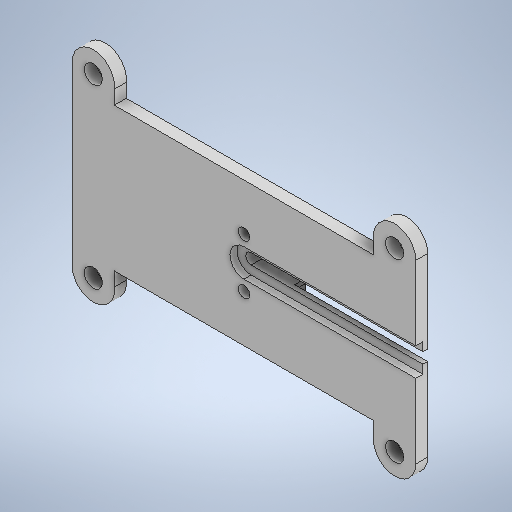
# Autodesk Inventor part: Gripper_BackPlate
Saved by Autodesk Inventor 2025.1 (Build 291241000, 241)
## iProperties
Created: 2024-08-02
Part Number: Gripper_BackPlate
Material: Generic
Document SubType Name: Modeling
Designer: leonh
Density: 1 g/cm^3
Appearance: Default
Author: leonh
Autodesk Inventor part; units mm, degrees
ref_plane "YZ Plane" through (0, 0, 0) normal (1, 0, 0) x (0, 1, 0)
ref_plane "XZ Plane" through (0, 0, 0) normal (0, 1, 0) x (-1, 0, 0)
ref_plane "XY Plane" through (0, 0, 0) normal (0, 0, 1) x (1, 0, 0)
sketch "Sketch1" plane through (0, 0, 0) normal (0, 0, 1) x (1, 0, 0)
  line L0 (-8.76, 11.0126) -> (-8.76, 0.5126)
  line L1 (-8.76, 0.5126) -> (-11.24, -14.9874)
  line L2 (-11.24, -14.9874) -> (8.76, -14.9874)
  line L3 (8.76, -14.9874) -> (8.76, -4.4874)
  line L4 (11.24, 11.0126) -> (-8.76, 11.0126)
  line L5 (0, 12.916) -> (0, -18.5653)
  line L6 (-8.76, 0.5126) -> (13.6474, 0.5126) construction
  line L7 (8.76, -4.4874) -> (-2.6872, -4.4874) construction
  line L8 (-5.8361, -1.9874) -> (18.6079, -1.9874) construction
  circle A0 centre (0, -7.7374) radius 1.325
  circle A1 centre (0, 3.7626) radius 1.325
  line L9 (22.7948, -1.9874) -> (0, -1.9874) construction
  line L10 (9.36, -0.7374) -> (0, -0.7374)
  line L11 (0, -3.2374) -> (8.96, -3.2374)
  arc A2 (0, -0.7374) -> (0, -3.2374) centre (0, -1.9874) ccw
  line L12 (8.76, -4.4874) -> (8.96, -3.2374)
  line L13 (9.36, -0.7374) -> (11.24, 11.0126)
  point P0 (0, 0)
  point P1 (-8.76, -4.4874)
  point P2 (11.3974, -1.9874)
  dimension "d0" = 2.48
  dimension "d1" = 15.5
  dimension "d2" = 15.5
  dimension "d3" = 2.48
  dimension "d4" = 10.5
  dimension "d5" = 10.5
  dimension "d6" = 20
  dimension "d7" = 20
  dimension "d8" = 2.65
  dimension "d9" = 7.25
  dimension "d12" = 2.5
  dimension "d26" = 11.75
  dimension "d27" = 14.25
  constraints: 30 end point, 4 point on line, 3 centre point, 2 horizontal, 2 perpendicular, 2 point on circle, 2 symmetric about line, 2 tangent, 2 vertical, 2 vertical alignment, 1 collinear, 1 midpoint, 1 parallel, 2 other
  measures "d0" horizontal distance of L1.end L0.end
  measures "d1" vertical distance of L1.end L0.end
  measures "d2" vertical distance of L4.start L3.end
  measures "d3" horizontal distance of L4.start L3.end
  measures "d4" distance of L0.start L0.end
  measures "d5" distance of L2.end L3.end
  measures "d6" distance of L4.start L0.start
  measures "d7" distance of L2.end L1.end
  measures "d8" diameter of A0
  measures "d9" distance from line of A0.centre L2
  measures "d12" diameter of A2
  measures "d26" vertical distance of L2.end L11.end
  measures "d27" vertical distance of L2.end L10.start
extrude "Extrusion1" add sketch "Sketch1" against normal blind 2.8 contours L4 L5 A1 A2 A0 L2 L1 L0 | L4 L13 L10 L5 A1 | L5 A0 L11 L12 L3 L2
sketch "Sketch2" plane through (0, 0, 0) normal (0, 0, 1) x (1, 0, 0)
  line L0 (-39.75, -18.5874) -> (-39.75, 14.6126)
  line L1 (0, 12.916) -> (0, -18.5653) construction
  line L2 (-5.8361, -1.9874) -> (18.6079, -1.9874) construction
  line L3 (-39.75, 14.6126) -> (-39.75, 18.4126)
  line L4 (-29.9847, 14.6126) -> (-29.9847, 17.8301)
  arc A0 (-29.9847, 17.8301) -> (-39.75, 18.4126) centre (-34.85, 18.4126) ccw
  line L5 (0, 12.916) -> (0, -18.5653)
  circle A1 centre (-34.85, 18.4126) radius 2.1
  arc A2 (0, -0.7374) -> (0, -3.2374) centre (0, -1.9874) ccw projected
  line L6 (-1.25, -1.9874) -> (17.7749, -1.9874) construction
  line L7 (0, -3.2374) -> (39.75, -3.2374)
  line L8 (39.75, -0.7374) -> (0, -0.7374)
  arc A3 (0, -0.7374) -> (0, -3.2374) centre (0, -1.9874) ccw
  line L9 (39.75, 14.6126) -> (39.75, -0.7374)
  line L10 (39.75, -3.2374) -> (39.75, -18.5874)
  line L11 (27.8114, -18.5874) -> (2.6919, -18.5874)
  line L12 (29.9847, -18.5874) -> (-29.9847, -18.5874)
  circle A4 centre (0, 3.7626) radius 1.325 projected
  circle A5 centre (0, -7.7374) radius 1.325 projected
  line L13 (-29.9847, 14.6126) -> (29.9847, 14.6126)
  line L14 (39.75, 14.6126) -> (39.75, 18.4126)
  line L15 (29.9847, 14.6126) -> (29.9847, 17.8301)
  arc A6 (39.75, 18.4126) -> (29.9847, 17.8301) centre (34.85, 18.4126) ccw
  circle A7 centre (34.85, 18.4126) radius 2.1
  line L16 (-39.75, -18.5874) -> (-39.75, -22.3874)
  line L17 (-29.9847, -18.5874) -> (-29.9847, -21.8049)
  arc A8 (-39.75, -22.3874) -> (-29.9847, -21.8049) centre (-34.85, -22.3874) ccw
  circle A9 centre (-34.85, -22.3874) radius 2.1
  line L18 (29.9847, -18.5874) -> (29.9847, -21.8049)
  circle A10 centre (34.85, -22.3874) radius 2.1
  line L19 (39.75, -18.5874) -> (39.75, -22.3874)
  arc A11 (29.9847, -21.8049) -> (39.75, -22.3874) centre (34.85, -22.3874) ccw
  point P0 (0, 0)
  point P1 (8.2624, -1.9874)
  point P2 (27.8114, 14.6126)
  dimension "d15" = 4.9
  dimension "d16" = 4.2
  dimension "d25" = 79.5
  constraints: 38 end point, 20 symmetric about line, 12 point on circle, 9 centre point, 5 point on line, 4 coincident, 3 parallel, 2 tangent, 2 vertical, 1 collinear, 1 horizontal, 1 midpoint, 1 vertical alignment, 7 other
  measures "d15" radius of A0
  measures "d16" diameter of A1
  measures "d25" distance between parallel lines of L0 L9
extrude "Extrusion2" add sketch "Sketch2" along normal blind 2.75 contours L0 L3 A0 L4 L13 L15 A6 L14 L9 L8 A2 L7 L10 L19 A11 L18 L12 L11 L17 A8 L16
sketch "Sketch3" plane through (0, 0, 2.75) normal (0, 0, 1) x (1, 0, 0)
  arc A0 (0, -0.7374) -> (0, -3.2374) centre (0, -1.9874) ccw projected
  line L0 (0, -1.9874) -> (45.1297, -1.9874) construction
  line L1 (0, -5.2374) -> (45.1297, -5.2374)
  line L2 (45.1297, 1.2626) -> (0, 1.2626)
  arc A1 (0, 1.2626) -> (0, -5.2374) centre (0, -1.9874) ccw
  arc A2 (45.1297, -5.2374) -> (45.1297, 1.2626) centre (45.1297, -1.9874) ccw
  point P0 (0, 0)
  point P1 (22.5649, -1.9874)
  dimension "d20" = 3.25
  constraints: 8 end point, 4 point on circle, 4 tangent, 2 centre point, 1 horizontal, 1 midpoint, 1 parallel
  measures "d20" radius of A1
extrude "Extrusion3" cut sketch "Sketch3" against normal blind 1.65
sketch "Sketch4" plane through (0, 0, 0) normal (0, 0, -1) x (-1, 0, 0)
  line L0 (-34.65, 8.0126) -> (-33.15, 8.0126)
  line L1 (-33.15, 8.0126) -> (-33.15, -0.7874)
  line L2 (-33.15, -0.7874) -> (-34.65, -0.7874)
  line L3 (-34.65, -0.7874) -> (-34.65, 8.0126)
  line L4 (-39.75, -0.7374) -> (-39.75, 18.4126) projected
  line L5 (-29.9847, 14.6126) -> (29.9847, 14.6126) projected
  line L6 (33.15, -3.1874) -> (34.65, -3.1874)
  line L7 (34.65, -3.1874) -> (34.65, -11.9874)
  line L8 (34.65, -11.9874) -> (33.15, -11.9874)
  line L9 (33.15, -11.9874) -> (33.15, -3.1874)
  line L10 (39.75, 18.4126) -> (39.75, -22.3874) projected
  line L11 (29.9847, -18.5874) -> (-29.9847, -18.5874) projected
  point P0 (0, 0)
  point P1 (-39.75, 8.8376)
  dimension "d28" = 5.1
  dimension "d29" = 6.6
  dimension "d30" = 8.8
  dimension "d31" = 1.5
  dimension "d32" = 5.1
  dimension "d33" = 6.6
  dimension "d34" = 8.8
  dimension "d35" = 1.5
  constraints: 16 end point, 4 parallel, 2 horizontal, 2 perpendicular, 1 midpoint
  measures "d28" distance from line of point (-39.75, 8.838) L3
  measures "d29" distance between parallel lines of L5 L0
  measures "d30" distance of L2.end L0.start
  measures "d31" distance between parallel lines of L1 L3
  measures "d32" distance between parallel lines of L10 L7
  measures "d33" distance between parallel lines of L11 L8
  measures "d34" distance between parallel lines of L8 L6
  measures "d35" distance between parallel lines of L7 L9
extrude "Extrusion4" add sketch "Sketch4" along normal blind 2.3
body "Solid1"
